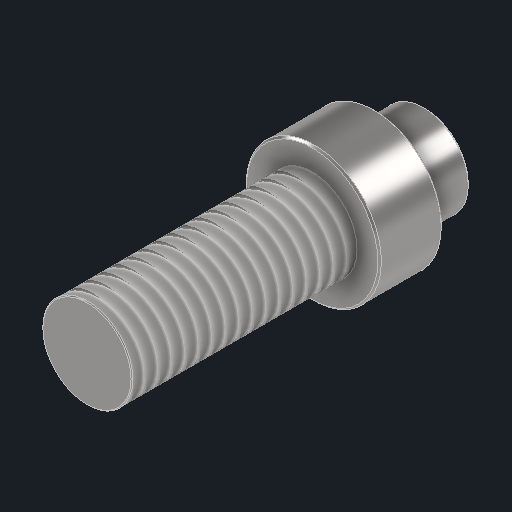
# Autodesk Inventor part: Pully Shaft
Saved by Autodesk Inventor 2027.1 (Build 311270010, 270A)
## iProperties
Created: 2025-09-16
Part Number: Pully Shaft
Material: Steel, Alloy
Document SubType Name: Modeling
Designer: SD
Density: 7.73 g/cm^3
Appearance: Semi-Polished
Mass: 26.2932 g
Surface Area: 18.1564 cm^2
Volume: 3.40145 cm^3
Project: Automatic Tea Steeping mechanism
Length: 37.550 mm
BOM-Mass: 0.02629
BOM-Area: 0.002
Diameter: 15.000 mm
Procurement: Fabricate - 1st round
Build Stage: 1
Preferred Material: Manufacturer Specification
Author: SD
Title: Pully Shaft
Autodesk Inventor part; units mm, degrees
ref_plane "YZ Plane" through (0, 0, 0) normal (1, 0, 0) x (0, 1, 0)
ref_plane "XZ Plane" through (0, 0, 0) normal (0, 1, 0) x (-1, 0, 0)
ref_plane "XY Plane" through (0, 0, 0) normal (0, 0, 1) x (1, 0, 0)
sketch "Sketch1" plane through (0, 0, 0) normal (0, 0, 1) x (1, 0, 0)
  circle A0 centre (0, 0) radius 7.5
  dimension "Diameter" = 15
  constraints: 1 centre point, 1 coincident
  measures "Diameter" diameter of A0
extrude "Extrusion1" add sketch "Sketch1" along normal blind 37.55
sketch "Sketch2" plane through (0, 0, 37.55) normal (0, 0, 1) x (1, 0, 0)
  circle A0 centre (0, 0) radius 5
  circle A1 centre (0, 0) radius 7.5 projected
  dimension "d3" = 10
  constraints: 1 centre point, 1 coincident
  measures "d3" diameter of A0
extrude "Extrusion2" cut sketch "Sketch2" against normal blind 25
chamfer "Chamfer1" distance 0.1 angle 45 1 edges at (-5, 0, 37.55)
thread "Thread1" size "M10x1.5" class "6g" standard "ANSI Metric M Profile" length 25
sketch "Sketch3" plane through (0, 0, 0) normal (0, 0, -1) x (-1, 0, 0)
  circle A0 centre (0, 0) radius 5
  circle A1 centre (0, 0) radius 7.5 projected
  dimension "d11" = 10
  constraints: 1 centre point, 1 coincident
  measures "d11" diameter of A0
extrude "Extrusion3" cut sketch "Sketch3" against normal blind 5.5
sketch "Sketch4" plane through (0, 0, 0) normal (0, 0, -1) x (-1, 0, 0)
  point P0 (0, 0)
  point P1 (0, 0)
  constraints: 1 coincident
hole "Hole1" at (0, 0, 0) direction (0, 0, 1) diameter 4.917 depth 12 tip angle 118 thread size "M6x1" class "6H" standard "ISO Metric profile"
chamfer "Chamfer2" distance 0.2 angle 45 3 edges at (5, 0, 0) (-7.5, 0, 5.5) (-7.5, 0, 12.55)
body "Solid1"
